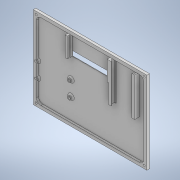
# Autodesk Inventor part: Back Cover v5
Saved by Autodesk Inventor 2021 (Build 250183000, 183)
## iProperties
Created: 2021-11-08
Part Number: Back Cover v5
Material: Generisch
Document SubType Name: Modeling
Designer: user
Density: 1 g/cm^3
Appearance: Vorgabe
Author: user
Autodesk Inventor part; units mm, degrees
ref_plane "YZ Plane" through (0, 0, 0) normal (1, 0, 0) x (0, 1, 0)
ref_plane "XY Plane" through (0, 0, 0) normal (0, 0, 1) x (1, 0, 0)
sketch "Skizze1" plane through (0, 0, 0) normal (0, 0, 1) x (1, 0, 0)
  line L0 (-90, -65.25) -> (90, -65.25)
  line L1 (90, -65.25) -> (90, 65.25)
  line L2 (90, 65.25) -> (-90, 65.25)
  line L3 (-90, 65.25) -> (-90, -65.25)
  line L4 (-90, -65.25) -> (90, 65.25) construction
  line L5 (90, -65.25) -> (-90, 65.25) construction
  point P0 (0, 0)
  dimension "d0" = 180
  dimension "d1" = 130.5
  constraints: 12 end point, 2 midpoint, 2 parallel, 1 horizontal, 1 perpendicular
  measures "d0" distance of L1.end L2.end
  measures "d1" distance of L2.end L0.start
extrude "Extrusion1" add sketch "Skizze1" along normal blind 0.8
sketch "Skizze2" plane through (0, 0, 0.8) normal (0, 0, 1) x (1, 0, 0)
  line L0 (90, -65.25) -> (90, 65.25) projected
  line L1 (90, 65.25) -> (-90, 65.25) projected
  line L2 (-90, 65.25) -> (-90, -65.25) projected
  line L3 (-90, -65.25) -> (90, -65.25) projected
  line L4 (-85, 60.25) -> (85, 60.25)
  line L5 (85, 60.25) -> (85, -60.25)
  line L6 (85, -60.25) -> (-85, -60.25)
  line L7 (-85, -60.25) -> (-85, 60.25)
  point P0 (0, 0)
  dimension "d4" = 5
  constraints: 8 end point, 3 other
  measures "d4" distance between parallel lines of L1 L4
extrude "Extrusion2" add sketch "Skizze2" along normal blind 3.2
ref_plane "Arbeitsebene1" through (0, 28.95, 0) normal (0, 1, 0) x (-1, 0, 0)
sketch "Skizze4" plane through (0, 28.95, 0) normal (0, 1, 0) x (-1, 0, 0)
  line L0 (0, 0) -> (0, 5.6907) construction
  line L1 (-85, 0.8) -> (85, 0.8) projected
  line L2 (31.5, 0.8) -> (35, 0.8)
  line L3 (35, 8.4503) -> (31.5, 8.4503)
  line L4 (35, 8.4503) -> (35, 0.8)
  line L5 (31.5, 8.4503) -> (31.5, 6.8503)
  line L6 (31.5, 6.8503) -> (33, 5.8)
  line L7 (33, 5.8) -> (31.5, 6.8503)
  line L8 (33, 5.8) -> (33, 4.2)
  line L9 (33, 4.2) -> (31.5, 4.2)
  line L10 (31.5, 4.2) -> (31.5, 0.8)
  line L11 (-90, 0) -> (90, 0) projected
  dimension "d8" = 33
  dimension "d9" = 1.6
  dimension "d11" = 125
  dimension "d12" = 1.5
  dimension "d13" = 1.6
  dimension "d14" = 2
  dimension "d17" = 4.2
  constraints: 20 end point, 3 perpendicular, 3 point on line, 3 vertical, 1 collinear, 1 horizontal
  measures "d8" distance between parallel lines of L0 L8
  measures "d9" distance of L6.end L8.end
  measures "d11" angle of L8 L6
  measures "d12" distance from line of L5 L6.end
  measures "d13" distance of L3.end L5.end
  measures "d14" distance between parallel lines of L4 L8
  measures "d17" distance between parallel lines of L11 L9
extrude "Extrusion3" add sketch "Skizze4" along normal up to surface (31.3 mm away)
sketch "Skizze5" plane through (-35, 60.25, 4) normal (0, 1, 0) x (1, 0, 0)
  line L0 (0, -4.4503) -> (3.5, -4.4503) projected
  line L1 (2, -0.2) -> (3.5, -0.2) projected
  line L2 (3.5, -4.4503) -> (3.5, -0.2)
  line L3 (3.5, -0.2) -> (0, -0.2)
  line L4 (0, 3.2) -> (0, -4.4503) projected
  line L5 (0, -0.2) -> (0, -4.4503)
  line L6 (0, -4.4503) -> (3.5, -4.4503)
  point P0 (35, 4)
  point P1 (0, -0.2)
  point P2 (0, 4.4503)
  point P3 (3.5, 4.4503)
  point P4 (2, 0.2)
  point P5 (3.5, 0.2)
  point P6 (0, 0)
  point P7 (0, -3.2)
  constraints: 8 end point, 1 collinear, 1 horizontal, 1 perpendicular, 1 vertical, 2 other
extrude "Extrusion4" add sketch "Skizze5" against normal blind 0.8
mirror "Spiegeln1" about plane through (0, 0, 0) normal (1, 0, 0) of "Extrusion3", "Extrusion4"
sketch "Skizze6" plane through (0, 0, 0.8) normal (0, 0, 1) x (1, 0, 0)
  line L0 (-31.5, 28.95) -> (-35, 28.95) projected
  line L1 (31.5, 28.95) -> (31.5, 60.25) projected
  line L2 (-31.5, 28.95) -> (31.5, 28.95)
  line L3 (31.5, 28.95) -> (31.5, 36.95)
  line L4 (31.5, 36.95) -> (-31.5, 36.95)
  line L5 (-31.5, 36.95) -> (-31.5, 28.95)
  point P0 (0, 0)
  dimension "d20" = 8
  constraints: 8 end point, 2 parallel, 1 horizontal, 1 perpendicular, 1 point on line
  measures "d20" distance between parallel lines of L2 L4
extrude "Extrusion5" cut sketch "Skizze6" against normal up to surface (0.8 mm away)
sketch "Skizze7" plane through (85, 60.25, 0.8) normal (0, -1, 0) x (1, 0, 0)
  line L0 (0, 0) -> (-50, 0) projected
  line L1 (-47.2, 0) -> (-47.2, 0.2)
  line L2 (-47.2, 0.2) -> (-49.6, 0.2)
  line L3 (-49.6, 0.2) -> (-49.6, 5.2)
  line L4 (5, 3.2) -> (-175, 3.2) projected
  line L5 (-49.6, 5.2) -> (-47.2, 6.8805)
  line L6 (-47.2, 6.8805) -> (-47.2, 7.6503)
  line L7 (-47.2, 7.6503) -> (-51.5, 7.6503)
  line L8 (-51.5, 7.6503) -> (-51.5, 0)
  line L9 (-51.5, 0) -> (-47.2, 0)
  line L10 (-50, 0) -> (-50, 7.6503) projected
  line L11 (-50, 7.6503) -> (-53.5, 7.6503) projected
  point P0 (-85, -0.8)
  point P1 (-50, 3.2)
  dimension "d23" = 0.2
  dimension "d24" = 5
  dimension "d25" = 125
  dimension "d26" = 2.4
  dimension "d31" = 1.5
  dimension "d32" = 0.4
  constraints: 16 end point, 3 collinear, 3 perpendicular, 2 point on line, 2 vertical
  measures "d23" distance of L1.start L1.end
  measures "d24" distance of L2.end L3.end
  measures "d25" angle of L3 L5
  measures "d26" distance of L1.end L2.end
  measures "d31" distance between parallel lines of L10 L8
  measures "d32" distance between parallel lines of L10 L3
extrude "Extrusion6" add sketch "Skizze7" along normal blind 61.2
ref_plane "Arbeitsebene2" through (54.2, 60.25, 6) normal (1, 0, 0) x (0, 0, -1)
mirror "Spiegeln2" about plane through (54.2, 60.25, 6) normal (1, 0, 0) of "Extrusion6"
sketch "Skizze8" plane through (0, 0, 0.8) normal (0, 0, 1) x (1, 0, 0)
  circle A0 centre (-86.5, -3.75) radius 3
  circle A1 centre (-33.4, -3.75) radius 3
  circle A2 centre (-33.4, -27.55) radius 3
  circle A3 centre (-86.5, -27.55) radius 3
  line L0 (-33.4, -27.55) -> (-33.4, -3.75) construction
  line L1 (-35, 28.95) -> (-35, 60.25) projected
  line L2 (-35, 28.95) -> (-35, -60.25) construction
  line L3 (85, -60.25) -> (-85, -60.25) projected
  line L4 (-33.4, -15.65) -> (-35, -15.65) construction
  line L5 (-90, 65.25) -> (-90, -65.25) projected
  point P0 (0, 0)
  dimension "d33" = 53.1
  dimension "d34" = 23.8
  dimension "d35" = 6
  dimension "d36" = 3.5
  constraints: 6 end point, 4 centre point, 3 equal radius, 2 horizontal alignment, 2 midpoint, 2 vertical, 2 vertical alignment, 1 perpendicular, 1 point on line
  measures "d33" distance of L0.end A0.centre
  measures "d34" distance of A3.centre A0.centre
  measures "d35" diameter of A0
  measures "d36" distance from line of L5 A3.centre
extrude "Extrusion7" add sketch "Skizze8" along normal blind 3.2
sketch "Skizze9" plane through (-33.4, -3.75, 4) normal (0, 0, 1) x (1, 0, 0)
  circle A0 centre (0, 0) radius 3 projected
  circle A1 centre (0, -23.8) radius 3 projected
  arc A2 (-51.6, -2.5981) -> (-51.6, 2.5981) centre (-53.1, 0) ccw projected
  arc A3 (-51.6, -26.3981) -> (-51.6, -21.2019) centre (-53.1, -23.8) ccw projected
  point P0 (33.4, 3.75)
hole "Bohrung1" at (-33.4, -3.75, 4) at (-33.4, -27.55, 4) at (-86.5, -3.75, 4) at (-86.5, -27.55, 4) direction (0, 0, -1) diameter 3.2 end through all
fillet "Rundung1" radius 2 4 edges at (-83.5, -3.75, 0.8) (-83.5, -27.55, 0.8) (-36.4, -27.55, 0.8) (-36.4, -3.75, 0.8)
fillet "Rundung2" radius 7 4 edges at (-85, 60.25, 2.4) (85, 60.25, 2.4) (85, -60.25, 2.4) (-85, -60.25, 2.4)
sketch "Skizze10" plane through (0, 0, 4) normal (0, 0, 1) x (1, 0, 0)
  line L0 (90, 65.25) -> (-90, 65.25) projected
  line L1 (-90, 65.25) -> (-90, -65.25) projected
  point P0 (0, 0)
  point P1 (-85.5, 60.75)
  dimension "d48" = 4.5
  dimension "d49" = 4.5
  measures "d48" distance from line of L0 point (-85.5, 60.75)
  measures "d49" distance from line of L1 point (-85.5, 60.75)
hole "Bohrung2" at (-85.5, 60.75, 4) direction (0, 0, -1) diameter 3.2 depth 15
mirror "Spiegeln3" about plane through (0, 0, 0) normal (1, 0, 0) of "Bohrung2"
mirror "Spiegeln4" about plane through (0, 0, 0) normal (0, 1, 0) of "Bohrung2", "Spiegeln3"
equation "\"d49\" = d48"
